Autodesk Fusion 360 part; units mm, degrees
note: some values were not read from the file. Chosen so that the rebuilt part matches the saved one: which bodies a step acts on; which face or edge a step refers to.
(part 2 of 2)
sketch "Skizze56" plane through (0, 0, 192.5) normal (0, 0, 1) x (-1, 0, 0)
  line L0 (38.6661, -111.8642) -> (38.6661, -129.3642)
  line L1 (38.6661, -129.3642) -> (3.6661, -129.3642)
  line L2 (3.6661, -129.3642) -> (3.6661, -111.8642)
  line L3 (3.6661, -111.8642) -> (38.6661, -111.8642)
  line L4 (41.2244, -132) -> (41.2244, -91.9905)
  line L5 (41.2244, -91.9905) -> (51.2244, -91.9905)
  line L6 (51.2244, -91.9905) -> (51.2244, -73.4478)
  line L7 (51.2244, -73.4478) -> (41.2244, -73.4478)
  line L8 (41.2244, -73.4478) -> (41.2244, -30)
  line L9 (41.2244, -30) -> (30.8999, -30)
  line L10 (30.8999, -30) -> (30.8999, -110)
  line L11 (30.8999, -110) -> (-61.0882, -110)
  line L12 (-61.0882, -110) -> (-61.0882, -30)
  line L13 (-61.0882, -30) -> (-70.2379, -30)
  line L14 (-70.2379, -30) -> (-70.0711, -104.5)
  line L15 (-70.0711, -104.5) -> (-70.0711, -113.1591)
  line L16 (-70.0711, -113.1591) -> (-17.2484, -113.1591)
  line L17 (-17.2484, -113.1591) -> (-17.2484, -113.2)
  line L18 (-17.2484, -113.2) -> (-17.3, -113.2)
  line L19 (-17.3, -113.2) -> (-17.3, -128.9)
  line L20 (-17.3, -128.9) -> (-17.2484, -128.9)
  line L21 (-17.2484, -128.9) -> (-17.2484, -129)
  line L22 (-17.2484, -129) -> (-70.0364, -129)
  line L23 (-70.0364, -129) -> (-70.0364, -130.5)
  line L24 (-70.0364, -130.5) -> (-70.0364, -132)
  line L25 (-70.0364, -132) -> (41.2244, -132)
hole "Bohrung3" at (-37.199, 111.8642, 188.5) direction (0, -1, 0) diameter 4 depth 35 tip angle 118 bodies 3
sketch "Skizze57" plane through (0, 89.2292, 0) normal (0, -1, 0) x (1, 0, 0)
  line L0 (-51.2244, 191) -> (-51.2244, 185.4)
  line L1 (-51.2244, 185.4) -> (-33.2244, 185.4)
  line L2 (-33.2244, 185.4) -> (-33.2244, 189.2548)
  line L3 (-33.2244, 189.2548) -> (-35, 190.25)
  line L4 (-35, 190.25) -> (-33.6333, 191)
  line L5 (-33.6333, 191) -> (-51.2244, 191)
  circle A0 centre (-37.199, 188.5) radius 2.1
sketch "Skizze58" plane through (-41.2244, 0, 0) normal (-1, 0, 0) x (0, -1, 0)
  line L0 (-132, 182.5) -> (-91.9905, 182.5)
  line L1 (-91.9905, 182.5) -> (-91.9905, 192.5)
  line L2 (-91.9905, 192.5) -> (-132, 192.5)
  line L3 (-132, 192.5) -> (-132, 182.5)
named bodies: "verteiler kappe", "tablat teil", "wand teil"
